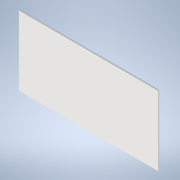
# Autodesk Inventor part: top
Saved by Autodesk Inventor 2021 (Build 250183000, 183)
## iProperties
Created: 2021-03-15
Part Number: top
Material: Všeobecné
Document SubType Name: Modeling
Designer: kanyk
Density: 1 g/cm^3
Appearance: Výchozí
Author: kanyk
Autodesk Inventor part; units mm, degrees
ref_plane "YZ Plane" through (0, 0, 0) normal (1, 0, 0) x (0, 1, 0)
ref_plane "XZ Plane" through (0, 0, 0) normal (0, 1, 0) x (-1, 0, 0)
ref_plane "XY Plane" through (0, 0, 0) normal (0, 0, 1) x (1, 0, 0)
sketch "Náčrt1" plane through (0, 0, 0) normal (0, 0, 1) x (1, 0, 0)
  line L0 (-48, 23) -> (48, 23) projected
  line L1 (48, 23) -> (48, -23) projected
  line L2 (48, -23) -> (-48, -23) projected
  line L3 (-48, -23) -> (-48, 23) projected
  line L4 (50, -25) -> (50, 25) projected
  line L5 (50, 25) -> (-50, 25) projected
  line L6 (-50, 25) -> (-50, -25) projected
  line L7 (-50, -25) -> (50, -25) projected
  line L8 (50, 25) -> (-50, 25) projected
  line L9 (50, 25) -> (-50, 25) projected
  line L10 (48, 23) -> (48, -23) projected
  line L11 (-48, 23) -> (48, 23) projected
  line L12 (-48, -23) -> (-48, 23) projected
  line L13 (48, -23) -> (-48, -23) projected
  point P0 (0, 0)
extrude "Vysunutí1" add sketch "Náčrt1" along normal blind 1
sketch "Náčrt2" plane through (0, 0, 1) normal (0, 0, 1) x (1, 0, 0)
  line L0 (-48, 23) -> (48, 23) projected
  line L1 (48, 23) -> (48, -23) projected
  line L2 (-48, 23) -> (48, 23) projected
  line L3 (-48, -23) -> (-48, 23) projected
  line L4 (48, -23) -> (-48, -23) projected
  point P0 (0, 0)
extrude "Vysunutí2" add sketch "Náčrt2" against normal blind 2
